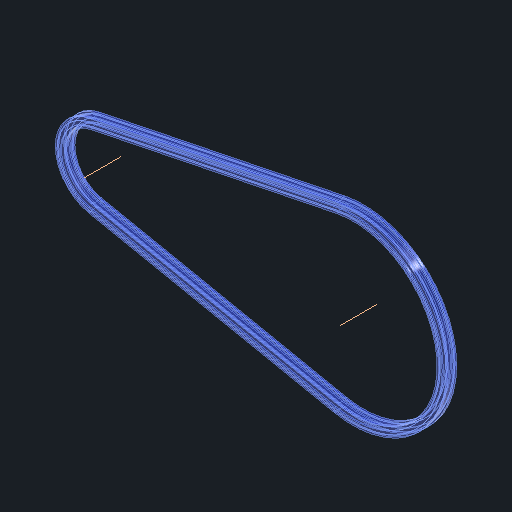
# Autodesk Inventor part: Roller Chain
Saved by Autodesk Inventor 2022 (Build 260153000, 153)
## iProperties
Created: 2023-01-04
Part Number: Roller Chain
Material: Generic
Document SubType Name: Modeling
Designer: HeavyDrewno
Density: 1 g/cm^3
Appearance: Clear - Blue
CustomPartVersion: 1
Author: HeavyDrewno
Autodesk Inventor part; units mm, degrees
ref_plane "Work Plane2" through (-133.0149, 0, 0) normal (-1, 0, 0) x (0, 0, 1)
ref_plane "Work Plane3" through (200, 0, 0) normal (-0.9814515, -0.1917106, 0) x (0, 0, 1)
sketch "Path" plane through (0, 0, 0) normal (0, 0, 1) x (1, 0, 0)
  arc A0 (-142.7475, 47.6658) -> (-142.7475, -47.6658) centre (-133.0149, 0) ccw
  arc A1 (176.9395, -112.9404) -> (176.9395, 112.9404) centre (200, 0) ccw
  line L0 (176.9395, -112.9404) -> (-142.7475, -47.6658)
  line L1 (-142.7475, 47.6658) -> (176.9395, 112.9404)
  dimension "d31" = 11.81
  constraints: 4 end point, 4 point on circle, 2 centre point
ref_plane "Section Plane" through (-142.7475, -47.6658, 0) normal (0.9797846, -0.2000552, 0) x (0, 0, 1)
sketch "Section Sketch" plane through (-142.7475, -47.6658, 0) normal (0.9797846, -0.2000552, 0) x (0, 0, 1)
  line L0 (-8.5, -2.225) -> (8.5, -2.225)
  line L1 (8.5, -2.225) -> (8.5, 2.225)
  line L2 (8.5, 2.225) -> (-8.5, 2.225)
  line L3 (-8.5, 2.225) -> (-8.5, -2.225)
  line L4 (-3.875, -4.255) -> (3.875, -4.255)
  line L5 (3.875, -4.255) -> (3.875, 4.255)
  line L6 (3.875, 4.255) -> (-3.875, 4.255)
  line L7 (-3.875, 4.255) -> (-3.875, -4.255)
  line L8 (-3.875, 0) -> (3.875, 0) construction
  line L9 (-6.875, -5.905) -> (-3.875, -5.905)
  line L10 (-3.875, -5.905) -> (-3.875, 5.905)
  line L11 (-3.875, 5.905) -> (-6.875, 5.905)
  line L12 (-6.875, 5.905) -> (-6.875, -5.905)
  line L13 (3.875, -5.905) -> (6.875, -5.905)
  line L14 (6.875, -5.905) -> (6.875, 5.905)
  line L15 (6.875, 5.905) -> (3.875, 5.905)
  line L16 (3.875, 5.905) -> (3.875, -5.905)
  line L17 (-8.5, 0) -> (8.5, 0) construction
  point P0 (0, 0)
  point P1 (0, 0)
  dimension "d21" = 4.45
  dimension "d22" = 8.51
  dimension "d23" = 7.75
  dimension "d24" = 3
  dimension "d31" = 11.81
  dimension "d32" = 17
  constraints: 36 end point, 8 midpoint, 8 parallel, 4 horizontal, 4 perpendicular, 3 collinear, 1 coincident, 1 other
  measures "d21" distance between parallel lines of L2 L0
  measures "d22" distance between parallel lines of L6 L4
  measures "d23" distance between parallel lines of L5 L7
  measures "d24" distance between parallel lines of L12 L10
  measures "d31" distance between parallel lines of L11 L9
  measures "d32" distance between parallel lines of L1 L3
sweep "Solid" add profiles "Section Sketch" path "Path"
pattern_of_one "Strand Pattern"
equation "\"d21\" = da_d2"
equation "\"d22\" = da_d1"
equation "\"d23\" = da_b1"
equation "\"d24\" = da_t1 + da_t2"
equation "\"d30\" = da_pt"
equation "\"da_p\" = 12.7"
equation "\"da_b1\" = 7.75"
equation "\"da_h2\" = 11.81"
equation "\"da_h3\" = 10.92"
equation "\"da_d1\" = 8.51"
equation "\"da_d2\" = 4.45"
equation "\"da_pt\" = 13.92"
equation "\"da_b\" = 17"
equation "\"da_t1\" = 1.5"
equation "\"da_t2\" = 1.5"
body "Solid1"
